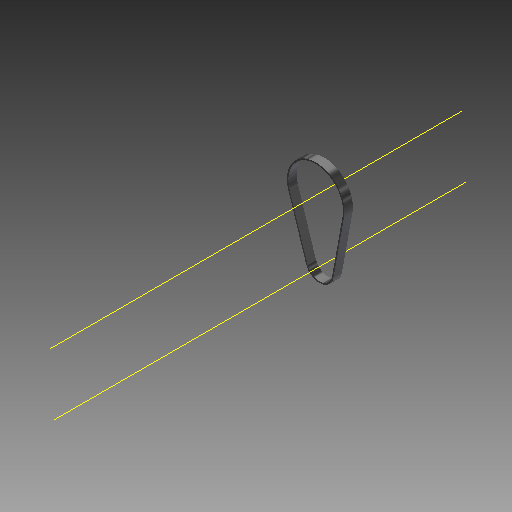
# Autodesk Inventor part: Synchronous Belt
Saved by Autodesk Inventor 2018.2 (Build 222227000, 227)
## iProperties
Created: 2018-02-12
Part Number: Synchronous Belt
Material: Rubber
Document SubType Name: Modeling
Designer: Moochster
Density: 1 g/cm^3
Appearance: Rubber - Black - Version 1.1
CustomPartVersion: 1
Author: Moochster
Autodesk Inventor part; units mm, degrees
ref_plane "YZ Plane" through (0, 0, 0) normal (1, 0, 0) x (0, 1, 0)
ref_plane "XZ Plane" through (0, 0, 0) normal (0, 1, 0) x (-1, 0, 0)
ref_plane "XY Plane" through (0, 0, 0) normal (0, 0, 1) x (1, 0, 0)
sketch "Sketch Path" plane through (0, 0, 0) normal (0, 0, 1) x (1, 0, 0)
  arc A0 (-6.372737, -45.310647) -> (12.112948, -44.124176) centre (2.721168, -42.396891) ccw
  arc A1 (19.56621, -3.598512) -> (-18.945634, -6.070325) centre (0, 0) ccw
  line L0 (19.56621, -3.598512) -> (12.112948, -44.124176)
  line L1 (-6.372737, -45.310647) -> (-18.945634, -6.070325)
  constraints: 4 end point, 2 point on circle, 1 centre point, 3 other
ref_plane "Cross Section Plane" through (12.112948, -44.124176, 0) normal (0.1808809, 0.983505, 0) x (0, 0, 1)
ref_plane "Work Plane2" through (2.721168, -42.396891, 0) normal (-1, 0, 0) x (0, 0, 1)
ref_plane "Work Plane3" through (0, 0, 0) normal (0.2200104, -0.9754975, 0) x (0, 0, 1)
sketch "Cross Section" plane through (12.112948, -44.124176, 0) normal (0.1808809, 0.983505, 0) x (0, 0, 1)
  line L0 (-3, 0.5) -> (3, 0.5)
  line L1 (3, 0.5) -> (3, -0.5)
  line L2 (3, -0.5) -> (-3, -0.5)
  line L3 (-3, -0.5) -> (-3, 0.5)
  line L4 (-3, 0) -> (3, 0) construction
  point P0 (0, 0)
  point P1 (0, 0)
  dimension "d0" = 6
  dimension "d4" = 0.5
  dimension "d5" = 0.5
  constraints: 10 end point, 3 midpoint, 2 parallel, 1 coincident, 1 horizontal, 1 perpendicular, 1 other
  measures "d0" distance between parallel lines of L1 L3
  measures "d4" distance between parallel lines of L2 L4
  measures "d5" distance between parallel lines of L4 L0
sweep "Belt" add profiles "Cross Section" path "Sketch Path" path curves L1 A1 L0 A0
equation "\"d0\" = da_B"
equation "\"d4\" = da_a"
equation "\"d5\" = da_a2"
equation "\"da_B\" = 6"
equation "\"da_pb\" = 5"
equation "\"da_a\" = 0.5"
equation "\"da_S\" = 2.65"
equation "\"da_Beta\" = 20deg"
equation "\"da_Ht\" = 1.2"
equation "\"da_H\" = 2.2"
equation "\"da_a2\" = 0.5"
body "Solid1"
